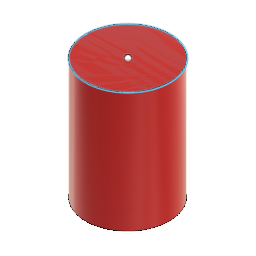
Pilon for Wheel with Spike (Autodesk Fusion 360 design; units mm, degrees)
Autodesk Fusion 360 part; units mm, degrees
sketch "sketch 347" plane through (0, 0, 3) normal (0, 0, 1) x (-1, 0, 0)
  circle A0 centre (-48.782, -46.5698) radius 12.5
  circle A1 centre (-48.782, -46.5698) radius 12.5
extrude "Extrude1" add sketch "sketch 347" against normal blind 36
extrude "Extrude2" cut 1 faces at (49.0934, 48.9301, -33) along direction (0, 0, 1) blind 8
extrude "Extrude3" add 1 faces at (49.0934, 48.9301, -25) along direction (0, 0, -1) blind 8
